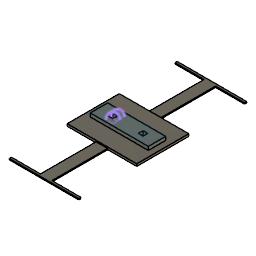
Ventillator Halterung (Autodesk Fusion 360 design; units mm, degrees)
part number: 2026-08-07-14-23-12-685
Autodesk Fusion 360 part; units mm, degrees
sketch "Sketch1" plane through (0, 0, 0) normal (0, 0, 1) x (1, 0, 0)
  line L0 (0, 0) -> (60, 0)
  line L1 (60, 0) -> (60, -25)
  line L2 (60, -25) -> (0, -25)
  line L3 (0, -25) -> (0, 0)
  line L4 (5, -5) -> (55, -5)
  line L5 (55, -5) -> (55, -20)
  line L6 (55, -20) -> (5, -20)
  line L7 (5, -20) -> (5, -5)
  line L8 (41, -10.5) -> (45, -10.5)
  line L9 (45, -10.5) -> (45, -14.5)
  line L10 (45, -14.5) -> (41, -14.5)
  line L11 (41, -14.5) -> (41, -10.5)
  line L12 (15, -10.5) -> (19, -10.5)
  line L13 (19, -10.5) -> (19, -14.5)
  line L14 (19, -14.5) -> (15, -14.5)
  line L15 (15, -14.5) -> (15, -10.5)
  dimension "d1" = 60
  dimension "d2" = 25
  dimension "d3" = 50
  dimension "d4" = 15
  dimension "d5" = 5
  dimension "d6" = 5
  dimension "d7" = 4
  dimension "d8" = 10
  dimension "d9" = 5.5
  dimension "d10" = 4
  dimension "d11" = 4
  dimension "d12" = 5.5
  dimension "d13" = 10
  dimension "d14" = 4
  constraint horizontal L0
  constraint vertical L1
  constraint horizontal L2
  constraint vertical L3
  constraint coincident L0.start L3.end
  constraint horizontal L4
  constraint vertical L5
  constraint horizontal L6
  constraint vertical L7
  constraint horizontal L8
  constraint vertical L9
  constraint horizontal L10
  constraint vertical L11
  constraint horizontal L12
  constraint vertical L13
  constraint horizontal L14
  constraint vertical L15
  measures "d1" distance of L0.start L0.end
  measures "d2" distance of L0.start L2.end
  measures "d3" distance of L4.start L4.end
  measures "d4" distance of L4.start L6.end
  measures "d5" distance of L3 L7
  measures "d6" distance of L2 L6
  measures "d7" distance of L8.start L10.end
  measures "d8" distance of L5 L9
  measures "d9" distance of L4 L8
  measures "d10" distance of L9 L11
  measures "d11" distance of L12.start L12.end
  measures "d12" distance of L4 L12
  measures "d13" distance of L7 L15
  measures "d14" distance of L12 L14
extrude "Extrude1" add sketch "Sketch1" along normal blind 2 contours L0 L1 L2 L3
sketch "Sketch2" plane through (0, 0, 0) normal (0, 0, 1) x (1, 0, 0)
  line L0 (15, -10.5) -> (19, -10.5)
  line L1 (19, -10.5) -> (19, -14.5)
  line L2 (19, -14.5) -> (15, -14.5)
  line L3 (15, -14.5) -> (15, -10.5)
  line L4 (41, -10.5) -> (45, -10.5)
  line L5 (45, -10.5) -> (45, -14.5)
  line L6 (45, -14.5) -> (41, -14.5)
  line L7 (41, -14.5) -> (41, -10.5)
  line L8 (55, -5) -> (55, -20)
  line L9 (55, -20) -> (5, -20)
  line L10 (5, -20) -> (5, -5)
  line L11 (5, -5) -> (55, -5)
  dimension "d17" = 4
  dimension "d18" = 10
  dimension "d19" = 5.5
  dimension "d20" = 4
  dimension "d21" = 4
  dimension "d22" = 10
  dimension "d23" = 5.5
  dimension "d24" = 4
  constraint horizontal L0
  constraint vertical L1
  constraint horizontal L2
  constraint vertical L3
  constraint horizontal L4
  constraint vertical L5
  constraint horizontal L6
  constraint vertical L7
  measures "d17" distance of L4.start L4.end
  measures "d18" distance of L5 L8
  measures "d19" distance of L6 L9
  measures "d20" distance of L4 L6
  measures "d21" distance of L0.start L2.end
  measures "d22" distance of L3 L10
  measures "d23" distance of L0 L11
  measures "d24" distance of L1 L3
extrude "Extrude2" add sketch "Sketch2" along normal blind 5
extrude "Extrude3" add 1 faces at (40, -25, 0.6667) along direction (0, -1, 0) blind 10
extrude "Extrude4" add 1 faces at (20, 0, 0.6667) along direction (0, 1, 0) blind 10
sketch "Sketch3" plane through (0, -35, 0) normal (0, -1, 0) x (1, 0, 0)
  line L0 (0, 0) -> (60, 0)
  line L1 (60, 0) -> (60, 2)
  line L2 (60, 2) -> (0, 2)
  line L3 (0, 2) -> (0, 0)
  line L4 (25, 0) -> (35, 0)
  line L5 (35, 0) -> (35, 1)
  line L6 (35, 1) -> (25, 1)
  line L7 (25, 1) -> (25, 0)
  line L8 (41, 0) -> (41, 5)
  dimension "d31" = 1
  dimension "d32" = 6
  dimension "d33" = 10
  constraint horizontal L4
  constraint vertical L5
  constraint horizontal L6
  constraint vertical L7
  constraint coincident L0 L4.start
  measures "d31" distance of L2 L6
  measures "d32" distance of L5 L8
  measures "d33" distance of L5 L7
extrude "Extrude5" add sketch "Sketch3" along normal blind 50 contours L0 L4 L5 L6 L7
sketch "Sketch4" plane through (0, 10, 0) normal (0, 1, 0) x (-1, 0, 0)
  line L0 (-60, 0) -> (0, 0)
  line L1 (0, 0) -> (0, 2)
  line L2 (0, 2) -> (-60, 2)
  line L3 (-60, 2) -> (-60, 0)
  line L4 (-35, 1) -> (-25, 1)
  line L5 (-25, 1) -> (-25, 0)
  line L6 (-25, 0) -> (-35, 0)
  line L7 (-35, 0) -> (-35, 1)
  line L8 (-19, 0) -> (-19, 5)
  line L9 (-41, 0) -> (-41, 5)
  dimension "d36" = 6
  dimension "d37" = 1
  dimension "d38" = 6
  constraint horizontal L4
  constraint vertical L5
  constraint horizontal L6
  constraint vertical L7
  constraint coincident L0 L5.end
  measures "d36" distance of L5 L8
  measures "d37" distance of L2 L4
  measures "d38" distance of L4.start L9
extrude "Extrude6" add sketch "Sketch4" along normal blind 50 contours L0 L4 L5 L6 L7
sketch "Sketch5" plane through (35, 0, 0) normal (1, 0, 0) x (0, 1, 0)
  line L0 (-35, 0) -> (-35, 1)
  line L1 (-35, 1) -> (-85, 1)
  line L2 (-85, 1) -> (-85, 0)
  line L3 (-85, 0) -> (-35, 0)
  line L4 (-85, 1) -> (-83, 1)
  line L5 (-83, 1) -> (-83, 0)
  line L6 (-83, 0) -> (-85, 0)
  line L7 (-85, 0) -> (-85, 1)
  dimension "d41" = 2
  constraint horizontal L4
  constraint vertical L5
  constraint horizontal L6
  constraint vertical L7
  constraint coincident L3 L5.end
  constraint coincident L1.end L2.start
  measures "d41" distance of L5 L7
extrude "Extrude7" add sketch "Sketch5" along normal blind 25 contours L1 L2 L3 L4 L5 L6 L7
sketch "Sketch6" plane through (25, 0, 0) normal (-1, 0, 0) x (0, -1, 0)
  line L0 (35, 1) -> (35, 0)
  line L1 (35, 0) -> (85, 0)
  line L2 (85, 0) -> (85, 1)
  line L3 (85, 1) -> (35, 1)
  line L4 (85, 0) -> (83, 0)
  line L5 (83, 0) -> (83, 1)
  line L6 (83, 1) -> (85, 1)
  line L7 (85, 1) -> (85, 0)
  dimension "d44" = 2
  constraint horizontal L4
  constraint vertical L5
  constraint horizontal L6
  constraint vertical L7
  constraint coincident L3 L5.end
  constraint coincident L1.end L2.start
  measures "d44" distance of L5 L7
extrude "Extrude8" add sketch "Sketch6" along normal blind 25 contours L1 L2 L3 L4 L5 L6 L7
sketch "Sketch7" plane through (25, 0, 0) normal (-1, 0, 0) x (0, -1, 0)
  line L0 (-10, 0) -> (-10, 1)
  line L1 (-10, 1) -> (-60, 1)
  line L2 (-60, 1) -> (-60, 0)
  line L3 (-60, 0) -> (-10, 0)
  line L4 (-60, 1) -> (-58, 1)
  line L5 (-58, 1) -> (-58, 0)
  line L6 (-58, 0) -> (-60, 0)
  line L7 (-60, 0) -> (-60, 1)
  dimension "d47" = 2
  constraint horizontal L4
  constraint vertical L5
  constraint horizontal L6
  constraint vertical L7
  constraint coincident L3 L5.end
  constraint coincident L1.end L2.start
  measures "d47" distance of L5 L7
extrude "Extrude9" add sketch "Sketch7" along normal blind 25 contours L1 L2 L3 L4 L5 L6 L7
sketch "Sketch8" plane through (35, 0, 0) normal (1, 0, 0) x (0, 1, 0)
  line L0 (10, 1) -> (10, 0)
  line L1 (10, 0) -> (60, 0)
  line L2 (60, 0) -> (60, 1)
  line L3 (60, 1) -> (10, 1)
  line L4 (58, 1) -> (60, 1)
  line L5 (60, 1) -> (60, 0)
  line L6 (60, 0) -> (58, 0)
  line L7 (58, 0) -> (58, 1)
  dimension "d50" = 2
  constraint horizontal L4
  constraint vertical L5
  constraint horizontal L6
  constraint vertical L7
  constraint coincident L1.end L2.start
  constraint coincident L3 L4.start
  measures "d50" distance of L5 L7
extrude "Extrude10" add sketch "Sketch8" along normal blind 25 contours L1 L2 L3 L4 L5 L6 L7
sketch "Sketch9" plane through (0, 0, 5) normal (0, 0, 1) x (-1, 0, 0)
  line L0 (-19, 14.5) -> (-15, 14.5)
  line L1 (-15, 14.5) -> (-15, 10.5)
  line L2 (-15, 10.5) -> (-19, 10.5)
  line L3 (-45, 14.5) -> (-41, 14.5)
  line L4 (-41, 14.5) -> (-41, 10.5)
  line L5 (-41, 10.5) -> (-45, 10.5)
  line L6 (-45, 10.5) -> (-45, 14.5)
  line L7 (-5, 5) -> (-5, 20)
  line L8 (-5, 20) -> (-55, 20)
  line L9 (-55, 20) -> (-55, 5)
  line L10 (-55, 5) -> (-5, 5)
